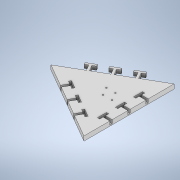
# Autodesk Inventor part: Base2
Saved by Autodesk Inventor 2022.3 (Build 263350000, 350)
## iProperties
Created: 2023-03-28
Part Number: Base2
Material: Generic
Document SubType Name: Modeling
Designer: Manuel Hueso Béjar
Density: 1 g/cm^3
Appearance: Default
Author: Manuel Hueso Béjar
Autodesk Inventor part; units mm, degrees
ref_plane "YZ Plane" through (0, 0, 0) normal (1, 0, 0) x (0, 1, 0)
ref_plane "XZ Plane" through (0, 0, 0) normal (0, 1, 0) x (-1, 0, 0)
ref_plane "XY Plane" through (0, 0, 0) normal (0, 0, 1) x (1, 0, 0)
sketch "Sketch1" plane through (0, 0, 0) normal (0, 1, 0) x (-1, 0, 0)
  circle A0 centre (0, 0) radius 115.470054
  line L0 (115.470054, 0) -> (-57.735027, -100)
  line L1 (-57.735027, -100) -> (-57.735027, 100)
  line L2 (-57.735027, 100) -> (115.470054, 0)
  line L3 (-40.235027, 2.5) -> (-75.235027, 2.5)
  line L4 (-75.235027, 2.5) -> (-75.235027, -2.5)
  line L5 (-75.235027, -2.5) -> (-40.235027, -2.5)
  line L6 (-40.235027, -2.5) -> (-40.235027, 2.5)
  line L7 (-40.235027, 2.5) -> (-75.235027, -2.5) construction
  line L8 (-75.235027, 2.5) -> (-40.235027, -2.5) construction
  line L9 (-42.735027, 10) -> (-37.735027, 10)
  line L10 (-37.735027, 10) -> (-37.735027, -10)
  line L11 (-37.735027, -10) -> (-42.735027, -10)
  line L12 (-42.735027, -10) -> (-42.735027, 10)
  line L13 (-42.735027, 10) -> (-37.735027, -10) construction
  line L14 (-37.735027, 10) -> (-42.735027, -10) construction
  line L15 (-37.735027, 50) -> (-37.735027, 30)
  line L16 (-42.735027, 50) -> (-37.735027, 50)
  line L17 (-42.735027, 30) -> (-42.735027, 50)
  line L18 (-37.735027, 30) -> (-42.735027, 30)
  line L19 (-40.235027, 42.5) -> (-75.235027, 42.5)
  line L20 (-75.235027, 37.5) -> (-40.235027, 37.5)
  line L21 (-37.735027, 90) -> (-37.735027, 70)
  line L22 (-42.735027, 90) -> (-37.735027, 90)
  line L23 (-42.735027, 70) -> (-42.735027, 90)
  line L24 (-37.735027, 70) -> (-42.735027, 70)
  line L25 (-40.235027, 82.5) -> (-75.235027, 82.5)
  line L26 (-75.235027, 77.5) -> (-40.235027, 77.5)
  line L27 (-37.735027, -30) -> (-37.735027, -50)
  line L28 (-42.735027, -30) -> (-37.735027, -30)
  line L29 (-42.735027, -50) -> (-42.735027, -30)
  line L30 (-37.735027, -50) -> (-42.735027, -50)
  line L31 (-40.235027, -37.5) -> (-75.235027, -37.5)
  line L32 (-75.235027, -42.5) -> (-40.235027, -42.5)
  line L33 (-37.735027, 10) -> (-37.735027, -10)
  line L34 (-42.735027, 10) -> (-37.735027, 10)
  line L35 (-42.735027, -10) -> (-42.735027, 10)
  line L36 (-37.735027, -10) -> (-42.735027, -10)
  line L37 (-40.235027, 2.5) -> (-75.235027, 2.5)
  line L38 (-75.235027, -2.5) -> (-40.235027, -2.5)
  line L39 (-37.735027, 50) -> (-37.735027, 30)
  line L40 (-42.735027, 50) -> (-37.735027, 50)
  line L41 (-42.735027, 30) -> (-42.735027, 50)
  line L42 (-37.735027, 30) -> (-42.735027, 30)
  line L43 (-40.235027, 42.5) -> (-75.235027, 42.5)
  line L44 (-75.235027, 37.5) -> (-40.235027, 37.5)
  line L45 (-37.735027, -70) -> (-37.735027, -90)
  line L46 (-42.735027, -70) -> (-37.735027, -70)
  line L47 (-42.735027, -90) -> (-42.735027, -70)
  line L48 (-37.735027, -90) -> (-42.735027, -90)
  line L49 (-40.235027, -77.5) -> (-75.235027, -77.5)
  line L50 (-75.235027, -82.5) -> (-40.235027, -82.5)
  line L51 (-37.735027, -30) -> (-37.735027, -50)
  line L52 (-42.735027, -30) -> (-37.735027, -30)
  line L53 (-42.735027, -50) -> (-42.735027, -30)
  line L54 (-37.735027, -50) -> (-42.735027, -50)
  line L55 (-40.235027, -37.5) -> (-75.235027, -37.5)
  line L56 (-75.235027, -42.5) -> (-40.235027, -42.5)
  line L57 (-37.735027, 10) -> (-37.735027, -10)
  line L58 (-42.735027, 10) -> (-37.735027, 10)
  line L59 (-42.735027, -10) -> (-42.735027, 10)
  line L60 (-37.735027, -10) -> (-42.735027, -10)
  line L61 (-40.235027, 2.5) -> (-75.235027, 2.5)
  line L62 (-75.235027, -2.5) -> (-40.235027, -2.5)
  point P0 (-57.735027, 0)
  point P1 (-40.235027, 0)
  point P2 (-42.735027, 42.5)
  point P3 (-57.735027, 42.5)
  point P4 (-57.735027, 37.5)
  point P5 (-42.735027, 37.5)
  point P6 (-42.735027, -37.5)
  point P7 (-57.735027, -37.5)
  point P8 (-57.735027, -42.5)
  point P9 (-42.735027, -42.5)
  point P10 (-42.735027, 82.5)
  point P11 (-57.735027, 82.5)
  point P12 (-57.735027, 77.5)
  point P13 (-42.735027, 77.5)
  point P14 (-42.735027, -77.5)
  point P15 (-57.735027, -77.5)
  point P16 (-57.735027, -82.5)
  point P17 (-42.735027, -82.5)
  point P18 (-42.735027, -2.5)
  point P19 (-42.735027, 2.5)
  point P20 (-57.735027, 2.5)
  point P21 (-57.735027, -2.5)
  point P22 (-40.414519, -90)
  point P23 (-37.735027, -88.452995)
  point P24 (-37.735027, 88.452995)
  point P25 (-40.414519, 90)
  dimension "d1" = 200
  dimension "d2" = 35
  dimension "d3" = 5
  dimension "d4" = 5
  dimension "d5" = 20
  dimension "d8" = 40
  dimension "d11" = 40
  constraints: 126 end point, 6 midpoint, 4 parallel, 2 coincident, 2 horizontal, 2 perpendicular, 2 vertical, 1 horizontal alignment, 121 other
  measures "d1" distance of L0.end L1.end
  measures "d2" distance of L5.end L4.end
  measures "d3" distance of L4.end L3.end
  measures "d4" distance of L10.end L11.end
  measures "d5" distance of L9.end L10.end
  measures "d8" distance of L9.end L15.start
  measures "d11" distance of L9.end L27.start
sketch "Sketch1 outline for Extrusion1" plane through (0, 0, 0) normal (0, 1, 0) x (-1, 0, 0)
  line L0 (-57.735027, 100) -> (-57.735027, -100)
  line L1 (115.470054, 0) -> (-57.735027, 100)
  line L2 (-57.735027, -100) -> (115.470054, 0)
extrude "Extrusion1" add sketch "Sketch1 outline for Extrusion1" along normal blind 10
sketch "Sketch1 outline for Extrusion2" plane through (0, 0, 0) normal (0, 1, 0) x (-1, 0, 0)
  line L0 (-42.735027, 30) -> (-37.735027, 30)
  line L1 (-42.735027, 37.5) -> (-42.735027, 30)
  line L2 (-57.735027, 37.5) -> (-42.735027, 37.5)
  line L3 (-57.735027, 42.5) -> (-57.735027, 37.5)
  line L4 (-42.735027, 42.5) -> (-57.735027, 42.5)
  line L5 (-42.735027, 50) -> (-42.735027, 42.5)
  line L6 (-37.735027, 50) -> (-42.735027, 50)
  line L7 (-37.735027, 30) -> (-37.735027, 50)
  line L8 (-42.735027, -50) -> (-37.735027, -50)
  line L9 (-42.735027, -42.5) -> (-42.735027, -50)
  line L10 (-57.735027, -42.5) -> (-42.735027, -42.5)
  line L11 (-57.735027, -37.5) -> (-57.735027, -42.5)
  line L12 (-42.735027, -37.5) -> (-57.735027, -37.5)
  line L13 (-42.735027, -30) -> (-42.735027, -37.5)
  line L14 (-37.735027, -30) -> (-42.735027, -30)
  line L15 (-37.735027, -50) -> (-37.735027, -30)
  line L16 (-42.735027, -2.5) -> (-42.735027, -10)
  line L17 (-57.735027, -2.5) -> (-42.735027, -2.5)
  line L18 (-57.735027, 2.5) -> (-57.735027, -2.5)
  line L19 (-42.735027, 2.5) -> (-57.735027, 2.5)
  line L20 (-42.735027, 10) -> (-42.735027, 2.5)
  line L21 (-37.735027, 10) -> (-42.735027, 10)
  line L22 (-37.735027, -10) -> (-37.735027, 10)
  line L23 (-42.735027, -10) -> (-37.735027, -10)
extrude "Extrusion2" cut sketch "Sketch1 outline for Extrusion2" along normal blind 10
sketch "Sketch1 outline for Extrusion3" plane through (0, 0, 0) normal (0, 1, 0) x (-1, 0, 0)
  line L0 (-42.735027, 30) -> (-37.735027, 30)
  line L1 (-42.735027, 37.5) -> (-42.735027, 30)
  line L2 (-57.735027, 37.5) -> (-42.735027, 37.5)
  line L3 (-57.735027, 42.5) -> (-57.735027, 37.5)
  line L4 (-42.735027, 42.5) -> (-57.735027, 42.5)
  line L5 (-42.735027, 50) -> (-42.735027, 42.5)
  line L6 (-37.735027, 50) -> (-42.735027, 50)
  line L7 (-37.735027, 30) -> (-37.735027, 50)
  line L8 (-42.735027, -50) -> (-37.735027, -50)
  line L9 (-42.735027, -42.5) -> (-42.735027, -50)
  line L10 (-57.735027, -42.5) -> (-42.735027, -42.5)
  line L11 (-57.735027, -37.5) -> (-57.735027, -42.5)
  line L12 (-42.735027, -37.5) -> (-57.735027, -37.5)
  line L13 (-42.735027, -30) -> (-42.735027, -37.5)
  line L14 (-37.735027, -30) -> (-42.735027, -30)
  line L15 (-37.735027, -50) -> (-37.735027, -30)
  line L16 (-42.735027, -2.5) -> (-42.735027, -10)
  line L17 (-57.735027, -2.5) -> (-42.735027, -2.5)
  line L18 (-57.735027, 2.5) -> (-57.735027, -2.5)
  line L19 (-42.735027, 2.5) -> (-57.735027, 2.5)
  line L20 (-42.735027, 10) -> (-42.735027, 2.5)
  line L21 (-37.735027, 10) -> (-42.735027, 10)
  line L22 (-37.735027, -10) -> (-37.735027, 10)
  line L23 (-42.735027, -10) -> (-37.735027, -10)
  line L24 (-37.735027, -70) -> (-42.735027, -70)
  line L25 (-37.735027, -88.452995) -> (-37.735027, -70)
  line L26 (-40.414519, -90) -> (-37.735027, -88.452995)
  line L27 (-42.735027, -90) -> (-40.414519, -90)
  line L28 (-42.735027, -82.5) -> (-42.735027, -90)
  line L29 (-57.735027, -82.5) -> (-42.735027, -82.5)
  line L30 (-57.735027, -77.5) -> (-57.735027, -82.5)
  line L31 (-42.735027, -77.5) -> (-57.735027, -77.5)
  line L32 (-42.735027, -70) -> (-42.735027, -77.5)
  line L33 (-42.735027, 70) -> (-37.735027, 70)
  line L34 (-42.735027, 77.5) -> (-42.735027, 70)
  line L35 (-57.735027, 77.5) -> (-42.735027, 77.5)
  line L36 (-57.735027, 82.5) -> (-57.735027, 77.5)
  line L37 (-42.735027, 82.5) -> (-57.735027, 82.5)
  line L38 (-42.735027, 90) -> (-42.735027, 82.5)
  line L39 (-40.414519, 90) -> (-42.735027, 90)
  line L40 (-37.735027, 88.452995) -> (-40.414519, 90)
  line L41 (-37.735027, 70) -> (-37.735027, 88.452995)
extrude "Extrusion3" add sketch "Sketch1 outline for Extrusion3" along normal blind 2.2
sketch "Sketch2" plane through (0, 0, 0) normal (0, -1, 0) x (1, 0, 0)
  line L0 (57.735027, 100) -> (57.735027, -100)
  line L1 (-115.470054, 0) -> (57.735027, 100)
  line L2 (57.735027, -100) -> (-115.470054, 0)
  line L3 (35.735027, 61.894882) -> (35.735027, -61.894882)
  line L4 (35.735027, -61.894882) -> (-71.470054, 0)
  line L5 (-71.470054, 0) -> (35.735027, 61.894882)
  line L6 (32.735027, 56.69873) -> (32.735027, -56.69873)
  line L7 (32.735027, -56.69873) -> (-65.470054, 0)
  line L8 (-65.470054, 0) -> (32.735027, 56.69873)
  point P0 (0, 0)
  dimension "d20" = 22
  dimension "d21" = 3
  constraints: 12 end point, 4 other
  measures "d20" distance between parallel lines of L1 L5
  measures "d21" distance between parallel lines of L5 L8
sketch "Sketch2 outline for Extrusion4" plane through (0, 0, 0) normal (0, -1, 0) x (1, 0, 0)
  line L0 (35.735027, 61.894882) -> (-71.470054, 0)
  line L1 (35.735027, -61.894882) -> (35.735027, 61.894882)
  line L2 (-71.470054, 0) -> (35.735027, -61.894882)
  line L3 (32.735027, 56.69873) -> (32.735027, -56.69873)
  line L4 (-65.470054, 0) -> (32.735027, 56.69873)
  line L5 (32.735027, -56.69873) -> (-65.470054, 0)
extrude "Extrusion4" cut sketch "Sketch2 outline for Extrusion4" against normal blind 1.5
sketch "Sketch3" plane through (0, 10, 0) normal (0, 1, 0) x (1, 0, 0)
  line L0 (57.735027, 100) -> (-115.470054, 0)
  line L1 (-28.867513, 50) -> (-36.367513, 62.990381)
  line L2 (-28.867513, 50) -> (-13.867513, 50) construction
  line L3 (-34.20245, 64.240381) -> (-27.707259, 67.990381)
  line L4 (-27.707259, 67.990381) -> (-30.207259, 72.320508)
  line L5 (-30.207259, 72.320508) -> (-47.527767, 62.320508)
  line L6 (-47.527767, 62.320508) -> (-45.027767, 57.990381)
  line L7 (-45.027767, 57.990381) -> (-38.532577, 61.740381)
  line L8 (-28.867513, 50) -> (-31.032577, 48.75)
  line L9 (-31.032577, 48.75) -> (-38.532577, 61.740381)
  line L10 (-31.032577, 48.75) -> (-26.70245, 51.25)
  line L11 (-26.70245, 51.25) -> (-34.20245, 64.240381)
  line L12 (-28.867513, -50) -> (-36.367513, -37.009619) construction
  line L13 (-28.867513, -50) -> (-26.70245, -51.25)
  line L14 (-26.70245, -51.25) -> (-31.032577, -48.75)
  line L15 (-28.867513, -50) -> (-36.367513, -62.990381)
  line L16 (-26.70245, -51.25) -> (-34.20245, -64.240381)
  line L17 (-31.032577, -48.75) -> (-38.532577, -61.740381)
  line L18 (-38.532577, -61.740381) -> (-45.027767, -57.990381)
  line L19 (-27.707259, -67.990381) -> (-34.20245, -64.240381)
  line L20 (-45.027767, -57.990381) -> (-47.527767, -62.320508)
  line L21 (-30.207259, -72.320508) -> (-27.707259, -67.990381)
  line L22 (-47.527767, -62.320508) -> (-30.207259, -72.320508)
  line L23 (-82.168784, 42.320508) -> (-79.668784, 37.990381)
  line L24 (-79.668784, 37.990381) -> (-73.173593, 41.740381)
  line L25 (-63.50853, 30) -> (-65.673593, 28.75)
  line L26 (-65.673593, 28.75) -> (-61.343466, 31.25)
  line L27 (-65.673593, 28.75) -> (-73.173593, 41.740381)
  line L28 (-63.50853, 30) -> (-71.00853, 42.990381)
  line L29 (-61.343466, 31.25) -> (-68.843466, 44.240381)
  line L30 (-64.848276, 52.320508) -> (-82.168784, 42.320508)
  line L31 (-63.50853, 30) -> (-48.50853, 30) construction
  line L32 (-62.348276, 47.990381) -> (-64.848276, 52.320508)
  line L33 (-68.843466, 44.240381) -> (-62.348276, 47.990381)
  line L34 (-116.8098, 22.320508) -> (-114.3098, 17.990381)
  line L35 (-114.3098, 17.990381) -> (-107.814609, 21.740381)
  line L36 (-98.149546, 10) -> (-100.314609, 8.75)
  line L37 (-100.314609, 8.75) -> (-95.984482, 11.25)
  line L38 (-100.314609, 8.75) -> (-107.814609, 21.740381)
  line L39 (-98.149546, 10) -> (-105.649546, 22.990381)
  line L40 (-95.984482, 11.25) -> (-103.484482, 24.240381)
  line L41 (-99.489292, 32.320508) -> (-116.8098, 22.320508)
  line L42 (-98.149546, 10) -> (-83.149546, 10) construction
  line L43 (-96.989292, 27.990381) -> (-99.489292, 32.320508)
  line L44 (-103.484482, 24.240381) -> (-96.989292, 27.990381)
  line L45 (-12.886751, 82.320508) -> (-10.386751, 77.990381)
  line L46 (-10.386751, 77.990381) -> (-3.891561, 81.740381)
  line L47 (5.773503, 70) -> (3.608439, 68.75)
  line L48 (3.608439, 68.75) -> (7.938566, 71.25)
  line L49 (3.608439, 68.75) -> (-3.891561, 81.740381)
  line L50 (5.773503, 70) -> (-1.726497, 82.990381)
  line L51 (7.938566, 71.25) -> (0.438566, 84.240381)
  line L52 (4.433757, 92.320508) -> (-12.886751, 82.320508)
  line L53 (5.773503, 70) -> (20.773503, 70) construction
  line L54 (6.933757, 87.990381) -> (4.433757, 92.320508)
  line L55 (0.438566, 84.240381) -> (6.933757, 87.990381)
  line L56 (-47.527767, 62.320508) -> (-45.027767, 57.990381)
  line L57 (-45.027767, 57.990381) -> (-38.532577, 61.740381)
  line L58 (-28.867513, 50) -> (-31.032577, 48.75)
  line L59 (-31.032577, 48.75) -> (-26.70245, 51.25)
  line L60 (-31.032577, 48.75) -> (-38.532577, 61.740381)
  line L61 (-28.867513, 50) -> (-36.367513, 62.990381)
  line L62 (-26.70245, 51.25) -> (-34.20245, 64.240381)
  line L63 (-30.207259, 72.320508) -> (-47.527767, 62.320508)
  line L64 (-28.867513, 50) -> (-13.867513, 50) construction
  line L65 (-27.707259, 67.990381) -> (-30.207259, 72.320508)
  line L66 (-34.20245, 64.240381) -> (-27.707259, 67.990381)
  line L67 (-82.168784, 42.320508) -> (-79.668784, 37.990381)
  line L68 (-79.668784, 37.990381) -> (-73.173593, 41.740381)
  line L69 (-63.50853, 30) -> (-65.673593, 28.75)
  line L70 (-65.673593, 28.75) -> (-61.343466, 31.25)
  line L71 (-65.673593, 28.75) -> (-73.173593, 41.740381)
  line L72 (-63.50853, 30) -> (-71.00853, 42.990381)
  line L73 (-61.343466, 31.25) -> (-68.843466, 44.240381)
  line L74 (-64.848276, 52.320508) -> (-82.168784, 42.320508)
  line L75 (-63.50853, 30) -> (-48.50853, 30) construction
  line L76 (-62.348276, 47.990381) -> (-64.848276, 52.320508)
  line L77 (-68.843466, 44.240381) -> (-62.348276, 47.990381)
  line L78 (21.754265, 102.320508) -> (24.254265, 97.990381)
  line L79 (24.254265, 97.990381) -> (30.749455, 101.740381)
  line L80 (40.414519, 90) -> (38.249455, 88.75)
  line L81 (38.249455, 88.75) -> (42.579582, 91.25)
  line L82 (38.249455, 88.75) -> (30.749455, 101.740381)
  line L83 (40.414519, 90) -> (32.914519, 102.990381)
  line L84 (42.579582, 91.25) -> (35.079582, 104.240381)
  line L85 (39.074773, 112.320508) -> (21.754265, 102.320508)
  line L86 (40.414519, 90) -> (55.414519, 90) construction
  line L87 (41.574773, 107.990381) -> (39.074773, 112.320508)
  line L88 (35.079582, 104.240381) -> (41.574773, 107.990381)
  line L89 (-12.886751, 82.320508) -> (-10.386751, 77.990381)
  line L90 (-10.386751, 77.990381) -> (-3.891561, 81.740381)
  line L91 (5.773503, 70) -> (3.608439, 68.75)
  line L92 (3.608439, 68.75) -> (7.938566, 71.25)
  line L93 (3.608439, 68.75) -> (-3.891561, 81.740381)
  line L94 (5.773503, 70) -> (-1.726497, 82.990381)
  line L95 (7.938566, 71.25) -> (0.438566, 84.240381)
  line L96 (4.433757, 92.320508) -> (-12.886751, 82.320508)
  line L97 (5.773503, 70) -> (20.773503, 70) construction
  line L98 (6.933757, 87.990381) -> (4.433757, 92.320508)
  line L99 (0.438566, 84.240381) -> (6.933757, 87.990381)
  line L100 (-47.527767, 62.320508) -> (-45.027767, 57.990381)
  line L101 (-45.027767, 57.990381) -> (-38.532577, 61.740381)
  line L102 (-28.867513, 50) -> (-31.032577, 48.75)
  line L103 (-31.032577, 48.75) -> (-26.70245, 51.25)
  line L104 (-31.032577, 48.75) -> (-38.532577, 61.740381)
  line L105 (-28.867513, 50) -> (-36.367513, 62.990381)
  line L106 (-26.70245, 51.25) -> (-34.20245, 64.240381)
  line L107 (-30.207259, 72.320508) -> (-47.527767, 62.320508)
  line L108 (-28.867513, 50) -> (-13.867513, 50) construction
  line L109 (-27.707259, 67.990381) -> (-30.207259, 72.320508)
  line L110 (-34.20245, 64.240381) -> (-27.707259, 67.990381)
  line L111 (-115.470054, 0) -> (57.735027, -100)
  line L112 (57.735027, -100) -> (-115.470054, 0)
  line L113 (5.773503, -70) -> (-1.726497, -57.009619) construction
  line L114 (5.773503, -70) -> (7.938566, -71.25)
  line L115 (7.938566, -71.25) -> (3.608439, -68.75)
  line L116 (3.608439, -68.75) -> (-3.891561, -81.740381)
  line L117 (5.773503, -70) -> (-1.726497, -82.990381)
  line L118 (7.938566, -71.25) -> (0.438566, -84.240381)
  line L119 (-3.891561, -81.740381) -> (-10.386751, -77.990381)
  line L120 (-10.386751, -77.990381) -> (-12.886751, -82.320508)
  line L121 (6.933757, -87.990381) -> (0.438566, -84.240381)
  line L122 (4.433757, -92.320508) -> (6.933757, -87.990381)
  line L123 (-12.886751, -82.320508) -> (4.433757, -92.320508)
  line L124 (40.414519, -90) -> (32.914519, -77.009619) construction
  line L125 (40.414519, -90) -> (42.579582, -91.25)
  line L126 (42.579582, -91.25) -> (38.249455, -88.75)
  line L127 (38.249455, -88.75) -> (30.749455, -101.740381)
  line L128 (40.414519, -90) -> (32.914519, -102.990381)
  line L129 (42.579582, -91.25) -> (35.079582, -104.240381)
  line L130 (30.749455, -101.740381) -> (24.254265, -97.990381)
  line L131 (24.254265, -97.990381) -> (21.754265, -102.320508)
  line L132 (41.574773, -107.990381) -> (35.079582, -104.240381)
  line L133 (39.074773, -112.320508) -> (41.574773, -107.990381)
  line L134 (21.754265, -102.320508) -> (39.074773, -112.320508)
  line L135 (-63.50853, -30) -> (-71.00853, -17.009619) construction
  line L136 (-63.50853, -30) -> (-61.343466, -31.25)
  line L137 (-61.343466, -31.25) -> (-65.673593, -28.75)
  line L138 (-65.673593, -28.75) -> (-73.173593, -41.740381)
  line L139 (-63.50853, -30) -> (-71.00853, -42.990381)
  line L140 (-61.343466, -31.25) -> (-68.843466, -44.240381)
  line L141 (-73.173593, -41.740381) -> (-79.668784, -37.990381)
  line L142 (-79.668784, -37.990381) -> (-82.168784, -42.320508)
  line L143 (-62.348276, -47.990381) -> (-68.843466, -44.240381)
  line L144 (-64.848276, -52.320508) -> (-62.348276, -47.990381)
  line L145 (-82.168784, -42.320508) -> (-64.848276, -52.320508)
  line L146 (-28.867513, -50) -> (-36.367513, -37.009619) construction
  line L147 (-28.867513, -50) -> (-26.70245, -51.25)
  line L148 (-26.70245, -51.25) -> (-31.032577, -48.75)
  line L149 (-31.032577, -48.75) -> (-38.532577, -61.740381)
  line L150 (-28.867513, -50) -> (-36.367513, -62.990381)
  line L151 (-26.70245, -51.25) -> (-34.20245, -64.240381)
  line L152 (-38.532577, -61.740381) -> (-45.027767, -57.990381)
  line L153 (-45.027767, -57.990381) -> (-47.527767, -62.320508)
  line L154 (-27.707259, -67.990381) -> (-34.20245, -64.240381)
  line L155 (-30.207259, -72.320508) -> (-27.707259, -67.990381)
  line L156 (-47.527767, -62.320508) -> (-30.207259, -72.320508)
  line L157 (5.773503, -70) -> (-1.726497, -57.009619) construction
  line L158 (5.773503, -70) -> (7.938566, -71.25)
  line L159 (7.938566, -71.25) -> (3.608439, -68.75)
  line L160 (3.608439, -68.75) -> (-3.891561, -81.740381)
  line L161 (5.773503, -70) -> (-1.726497, -82.990381)
  line L162 (7.938566, -71.25) -> (0.438566, -84.240381)
  line L163 (-3.891561, -81.740381) -> (-10.386751, -77.990381)
  line L164 (-10.386751, -77.990381) -> (-12.886751, -82.320508)
  line L165 (6.933757, -87.990381) -> (0.438566, -84.240381)
  line L166 (4.433757, -92.320508) -> (6.933757, -87.990381)
  line L167 (-12.886751, -82.320508) -> (4.433757, -92.320508)
  line L168 (-98.149546, -10) -> (-105.649546, 2.990381) construction
  line L169 (-98.149546, -10) -> (-95.984482, -11.25)
  line L170 (-95.984482, -11.25) -> (-100.314609, -8.75)
  line L171 (-100.314609, -8.75) -> (-107.814609, -21.740381)
  line L172 (-98.149546, -10) -> (-105.649546, -22.990381)
  line L173 (-95.984482, -11.25) -> (-103.484482, -24.240381)
  line L174 (-107.814609, -21.740381) -> (-114.3098, -17.990381)
  line L175 (-114.3098, -17.990381) -> (-116.8098, -22.320508)
  line L176 (-96.989292, -27.990381) -> (-103.484482, -24.240381)
  line L177 (-99.489292, -32.320508) -> (-96.989292, -27.990381)
  line L178 (-116.8098, -22.320508) -> (-99.489292, -32.320508)
  line L179 (-63.50853, -30) -> (-71.00853, -17.009619) construction
  line L180 (-63.50853, -30) -> (-61.343466, -31.25)
  line L181 (-61.343466, -31.25) -> (-65.673593, -28.75)
  line L182 (-65.673593, -28.75) -> (-73.173593, -41.740381)
  line L183 (-63.50853, -30) -> (-71.00853, -42.990381)
  line L184 (-61.343466, -31.25) -> (-68.843466, -44.240381)
  line L185 (-73.173593, -41.740381) -> (-79.668784, -37.990381)
  line L186 (-79.668784, -37.990381) -> (-82.168784, -42.320508)
  line L187 (-62.348276, -47.990381) -> (-68.843466, -44.240381)
  line L188 (-64.848276, -52.320508) -> (-62.348276, -47.990381)
  line L189 (-82.168784, -42.320508) -> (-64.848276, -52.320508)
  line L190 (-28.867513, -50) -> (-36.367513, -37.009619) construction
  line L191 (-28.867513, -50) -> (-26.70245, -51.25)
  line L192 (-26.70245, -51.25) -> (-31.032577, -48.75)
  line L193 (-31.032577, -48.75) -> (-38.532577, -61.740381)
  line L194 (-28.867513, -50) -> (-36.367513, -62.990381)
  line L195 (-26.70245, -51.25) -> (-34.20245, -64.240381)
  line L196 (-38.532577, -61.740381) -> (-45.027767, -57.990381)
  line L197 (-45.027767, -57.990381) -> (-47.527767, -62.320508)
  line L198 (-27.707259, -67.990381) -> (-34.20245, -64.240381)
  line L199 (-30.207259, -72.320508) -> (-27.707259, -67.990381)
  line L200 (-47.527767, -62.320508) -> (-30.207259, -72.320508)
  line L201 (-28.867513, -50) -> (-43.867513, -50) construction
  line L202 (-28.867513, -50) -> (-21.367513, -37.009619)
  line L203 (-26.70245, -51.25) -> (-19.20245, -38.259619)
  line L204 (-31.032577, -48.75) -> (-23.532577, -35.759619)
  line L205 (-23.532577, -35.759619) -> (-30.027767, -32.009619)
  line L206 (-12.707259, -42.009619) -> (-19.20245, -38.259619)
  line L207 (-30.027767, -32.009619) -> (-27.527767, -27.679492)
  line L208 (-10.207259, -37.679492) -> (-12.707259, -42.009619)
  line L209 (-27.527767, -27.679492) -> (-10.207259, -37.679492)
  line L210 (5.773503, -70) -> (-9.226497, -70) construction
  line L211 (3.608439, -68.75) -> (11.108439, -55.759619)
  line L212 (5.773503, -70) -> (13.273503, -57.009619)
  line L213 (7.938566, -71.25) -> (15.438566, -58.259619)
  line L214 (11.108439, -55.759619) -> (4.613249, -52.009619)
  line L215 (4.613249, -52.009619) -> (7.113249, -47.679492)
  line L216 (21.933757, -62.009619) -> (15.438566, -58.259619)
  line L217 (24.433757, -57.679492) -> (21.933757, -62.009619)
  line L218 (7.113249, -47.679492) -> (24.433757, -57.679492)
  line L219 (40.414519, -90) -> (25.414519, -90) construction
  line L220 (38.249455, -88.75) -> (45.749455, -75.759619)
  line L221 (40.414519, -90) -> (47.914519, -77.009619)
  line L222 (42.579582, -91.25) -> (50.079582, -78.259619)
  line L223 (45.749455, -75.759619) -> (39.254265, -72.009619)
  line L224 (39.254265, -72.009619) -> (41.754265, -67.679492)
  line L225 (56.574773, -82.009619) -> (50.079582, -78.259619)
  line L226 (59.074773, -77.679492) -> (56.574773, -82.009619)
  line L227 (41.754265, -67.679492) -> (59.074773, -77.679492)
  line L228 (-63.50853, -30) -> (-78.50853, -30) construction
  line L229 (-65.673593, -28.75) -> (-58.173593, -15.759619)
  line L230 (-63.50853, -30) -> (-56.00853, -17.009619)
  line L231 (-61.343466, -31.25) -> (-53.843466, -18.259619)
  line L232 (-58.173593, -15.759619) -> (-64.668784, -12.009619)
  line L233 (-64.668784, -12.009619) -> (-62.168784, -7.679492)
  line L234 (-47.348276, -22.009619) -> (-53.843466, -18.259619)
  line L235 (-44.848276, -17.679492) -> (-47.348276, -22.009619)
  line L236 (-62.168784, -7.679492) -> (-44.848276, -17.679492)
  line L237 (-28.867513, -50) -> (-43.867513, -50) construction
  line L238 (-31.032577, -48.75) -> (-23.532577, -35.759619)
  line L239 (-28.867513, -50) -> (-21.367513, -37.009619)
  line L240 (-26.70245, -51.25) -> (-19.20245, -38.259619)
  line L241 (-23.532577, -35.759619) -> (-30.027767, -32.009619)
  line L242 (-30.027767, -32.009619) -> (-27.527767, -27.679492)
  line L243 (-12.707259, -42.009619) -> (-19.20245, -38.259619)
  line L244 (-10.207259, -37.679492) -> (-12.707259, -42.009619)
  line L245 (-27.527767, -27.679492) -> (-10.207259, -37.679492)
  line L246 (5.773503, -70) -> (-9.226497, -70) construction
  line L247 (3.608439, -68.75) -> (11.108439, -55.759619)
  line L248 (5.773503, -70) -> (13.273503, -57.009619)
  line L249 (7.938566, -71.25) -> (15.438566, -58.259619)
  line L250 (11.108439, -55.759619) -> (4.613249, -52.009619)
  line L251 (4.613249, -52.009619) -> (7.113249, -47.679492)
  line L252 (21.933757, -62.009619) -> (15.438566, -58.259619)
  line L253 (24.433757, -57.679492) -> (21.933757, -62.009619)
  line L254 (7.113249, -47.679492) -> (24.433757, -57.679492)
  line L255 (-98.149546, -10) -> (-113.149546, -10) construction
  line L256 (-100.314609, -8.75) -> (-92.814609, 4.240381)
  line L257 (-98.149546, -10) -> (-90.649546, 2.990381)
  line L258 (-95.984482, -11.25) -> (-88.484482, 1.740381)
  line L259 (-92.814609, 4.240381) -> (-99.3098, 7.990381)
  line L260 (-99.3098, 7.990381) -> (-96.8098, 12.320508)
  line L261 (-81.989292, -2.009619) -> (-88.484482, 1.740381)
  line L262 (-79.489292, 2.320508) -> (-81.989292, -2.009619)
  line L263 (-96.8098, 12.320508) -> (-79.489292, 2.320508)
  line L264 (-63.50853, -30) -> (-78.50853, -30) construction
  line L265 (-65.673593, -28.75) -> (-58.173593, -15.759619)
  line L266 (-63.50853, -30) -> (-56.00853, -17.009619)
  line L267 (-61.343466, -31.25) -> (-53.843466, -18.259619)
  line L268 (-58.173593, -15.759619) -> (-64.668784, -12.009619)
  line L269 (-64.668784, -12.009619) -> (-62.168784, -7.679492)
  line L270 (-47.348276, -22.009619) -> (-53.843466, -18.259619)
  line L271 (-44.848276, -17.679492) -> (-47.348276, -22.009619)
  line L272 (-62.168784, -7.679492) -> (-44.848276, -17.679492)
  line L273 (-28.867513, -50) -> (-43.867513, -50) construction
  line L274 (-31.032577, -48.75) -> (-23.532577, -35.759619)
  line L275 (-28.867513, -50) -> (-21.367513, -37.009619)
  line L276 (-26.70245, -51.25) -> (-19.20245, -38.259619)
  line L277 (-23.532577, -35.759619) -> (-30.027767, -32.009619)
  line L278 (-30.027767, -32.009619) -> (-27.527767, -27.679492)
  line L279 (-12.707259, -42.009619) -> (-19.20245, -38.259619)
  line L280 (-10.207259, -37.679492) -> (-12.707259, -42.009619)
  line L281 (-27.527767, -27.679492) -> (-10.207259, -37.679492)
  point P0 (0, 0)
  point P1 (3.608439, 68.75)
  point P2 (7.938566, 71.25)
  point P3 (-65.673593, 28.75)
  point P4 (-61.343466, 31.25)
  point P5 (-100.314609, 8.75)
  point P6 (-95.984482, 11.25)
  point P7 (42.579582, -91.25)
  point P8 (38.249455, -88.75)
  point P9 (7.938566, -71.25)
  point P10 (3.608439, -68.75)
  point P11 (-61.343466, -31.25)
  point P12 (-65.673593, -28.75)
  point P13 (-95.984482, -11.25)
  point P14 (-100.314609, -8.75)
  point P15 (7.938566, -71.25)
  point P16 (3.608439, -68.75)
  point P17 (-12.707259, -42.009619)
  point P18 (-65.673593, -28.75)
  point P19 (-61.343466, -31.25)
  dimension "d24" = 15
  dimension "d25" = 120
  dimension "d26" = 10
  dimension "d27" = 5
  dimension "d28" = 20
  dimension "d29" = 90
  dimension "d30" = 5
  dimension "d31" = 2.5
  dimension "d32" = 5
  dimension "d35" = 120
  dimension "d39" = 40
  dimension "d42" = 40
  dimension "d47" = 40
  dimension "d50" = 40
  constraints: 560 end point, 72 symmetric about line, 6 perpendicular, 2 point on line, 1 collinear, 1 equal length, 1 horizontal, 1 midpoint, 379 other
  measures "d24" distance of L1.start L1.end
  measures "d25" angle of L2 L1
  measures "d26" distance of L1.end L3.end
  measures "d27" distance of L3.end L4.end
  measures "d28" distance of L4.end L5.end
  measures "d29" angle of L5 L4
  measures "d30" distance of L5.end L6.end
  measures "d31" distance of L1.start L8.end
  measures "d32" distance of L8.end L10.end
  measures "d39" distance of L6.end L23.end
  measures "d42" distance of L6.end L45.end
  measures "d47" distance of L12.end L113.end
  measures "d50" distance of L12.end L135.end
sketch "Sketch3 outline for Extrusion6" plane through (0, 10, 0) normal (0, 1, 0) x (1, 0, 0)
  line L0 (7.938566, -71.25) -> (15.438566, -58.259619)
  line L1 (3.608439, -68.75) -> (7.938566, -71.25)
  line L2 (11.108439, -55.759619) -> (3.608439, -68.75)
  line L3 (4.613249, -52.009619) -> (11.108439, -55.759619)
  line L4 (7.113249, -47.679492) -> (4.613249, -52.009619)
  line L5 (24.433757, -57.679492) -> (7.113249, -47.679492)
  line L6 (21.933757, -62.009619) -> (24.433757, -57.679492)
  line L7 (15.438566, -58.259619) -> (21.933757, -62.009619)
  line L8 (-10.207259, -37.679492) -> (-27.527767, -27.679492)
  line L9 (-27.527767, -27.679492) -> (-30.027767, -32.009619)
  line L10 (-30.027767, -32.009619) -> (-23.532577, -35.759619)
  line L11 (-23.532577, -35.759619) -> (-31.032577, -48.75)
  line L12 (-31.032577, -48.75) -> (-26.70245, -51.25)
  line L13 (-26.70245, -51.25) -> (-19.20245, -38.259619)
  line L14 (-19.20245, -38.259619) -> (-12.707259, -42.009619)
  line L15 (-12.707259, -42.009619) -> (-10.207259, -37.679492)
  line L16 (-44.848276, -17.679492) -> (-62.168784, -7.679492)
  line L17 (-47.348276, -22.009619) -> (-44.848276, -17.679492)
  line L18 (-53.843466, -18.259619) -> (-47.348276, -22.009619)
  line L19 (-61.343466, -31.25) -> (-53.843466, -18.259619)
  line L20 (-65.673593, -28.75) -> (-61.343466, -31.25)
  line L21 (-58.173593, -15.759619) -> (-65.673593, -28.75)
  line L22 (-64.668784, -12.009619) -> (-58.173593, -15.759619)
  line L23 (-62.168784, -7.679492) -> (-64.668784, -12.009619)
extrude "Extrusion6" cut sketch "Sketch3 outline for Extrusion6" against normal blind 7.8
sketch "Sketch3 outline for Extrusion7" plane through (0, 10, 0) normal (0, 1, 0) x (1, 0, 0)
  line L0 (0.438566, 84.240381) -> (6.933757, 87.990381)
  line L1 (7.938566, 71.25) -> (0.438566, 84.240381)
  line L2 (3.608439, 68.75) -> (7.938566, 71.25)
  line L3 (-3.891561, 81.740381) -> (3.608439, 68.75)
  line L4 (-10.386751, 77.990381) -> (-3.891561, 81.740381)
  line L5 (-12.886751, 82.320508) -> (-10.386751, 77.990381)
  line L6 (4.433757, 92.320508) -> (-12.886751, 82.320508)
  line L7 (6.933757, 87.990381) -> (4.433757, 92.320508)
  line L8 (-26.70245, 51.25) -> (-34.20245, 64.240381)
  line L9 (-31.032577, 48.75) -> (-26.70245, 51.25)
  line L10 (-38.532577, 61.740381) -> (-31.032577, 48.75)
  line L11 (-45.027767, 57.990381) -> (-38.532577, 61.740381)
  line L12 (-47.527767, 62.320508) -> (-45.027767, 57.990381)
  line L13 (-30.207259, 72.320508) -> (-47.527767, 62.320508)
  line L14 (-27.707259, 67.990381) -> (-30.207259, 72.320508)
  line L15 (-34.20245, 64.240381) -> (-27.707259, 67.990381)
  line L16 (-68.843466, 44.240381) -> (-62.348276, 47.990381)
  line L17 (-61.343466, 31.25) -> (-68.843466, 44.240381)
  line L18 (-65.673593, 28.75) -> (-61.343466, 31.25)
  line L19 (-73.173593, 41.740381) -> (-65.673593, 28.75)
  line L20 (-79.668784, 37.990381) -> (-73.173593, 41.740381)
  line L21 (-82.168784, 42.320508) -> (-79.668784, 37.990381)
  line L22 (-64.848276, 52.320508) -> (-82.168784, 42.320508)
  line L23 (-62.348276, 47.990381) -> (-64.848276, 52.320508)
extrude "Extrusion7" add sketch "Sketch3 outline for Extrusion7" against normal up to surface (7.8 mm away)
sketch "Sketch4" plane through (0, 10, 0) normal (0, 1, 0) x (1, 0, 0)
  line L0 (-115.470054, 0) -> (57.735027, 0)
  line L1 (57.735027, -100) -> (57.735027, 100)
  line L2 (57.735027, -100) -> (-28.867513, 50)
  line L3 (57.735027, 100) -> (-115.470054, 0)
  line L4 (57.735027, 100) -> (-28.867513, -50)
  line L5 (-115.470054, 0) -> (57.735027, -100)
  circle A0 centre (0, 0) radius 20
  line L6 (10, 17.320508) -> (20, 0)
  line L7 (20, 0) -> (10, -17.320508)
  line L8 (10, -17.320508) -> (-10, -17.320508)
  line L9 (-10, -17.320508) -> (-20, 0)
  line L10 (-20, 0) -> (-10, 17.320508)
  line L11 (-10, 17.320508) -> (10, 17.320508)
  dimension "d59" = 40
  constraints: 18 end point, 3 midpoint, 2 coincident, 1 point on line, 16 other
hole "Hole1" at (0, 10, 0) at (-10, 10, -17.320508) at (20, 10, 0) at (10, 10, -17.320508) direction (0, -1, 0) diameter 2.2 depth 6.3 counterbore diameter 3.1 counterbore depth 4.1
thicken "Thicken1" operation add thickness 0.05 both sides no extend neighbours yes toward (-0.8660254, 0, -0.5) faces at (-60.673593, 4.8, 20.089746) (-62.50372, 7.4, 13.259619) (-63.002117, 7.4, 9.122868) (-50.621778, 7.4, 14.346159) (-46.514942, 7.4, 20.566243) (-51.678403, 7.4, 19.509619) (-58.843466, 4.8, 26.919873)
thicken "Thicken2" operation add thickness 0.05 both sides no extend neighbours yes toward (-0.8660254, 0, -0.5) faces at (-26.032577, 7.4, 40.089746) (-27.862704, 7.4, 33.259619) (-28.361101, 7.4, 29.122868) (-15.980762, 4.8, 34.346159) (-11.040593, 4.8, 39.122868) (-17.037386, 7.4, 39.509619) (-24.20245, 4.8, 46.919873)
thicken "Thicken3" operation add thickness 0.05 both sides no extend neighbours yes toward (-0.8660254, 0, -0.5) faces at (6.108439, 4.8, 64.419873) (8.943376, 7.4, 54.509619) (6.279915, 7.4, 49.122868) (18.660254, 7.4, 54.346159) (22.76709, 7.4, 60.566243) (17.60363, 7.4, 59.509619) (10.438566, 7.4, 66.919873)
thicken "Thicken4" operation add thickness 0.05 both sides no extend neighbours yes toward (0, 0, 1) faces at (47.735027, 4.8, 42.5) (42.735027, 7.4, 47.5) (39.401694, 4.8, 50) (37.735027, 4.8, 36.666667) (41.06836, 4.8, 30) (42.735027, 7.4, 35) (52.735027, 4.8, 37.5)
thicken "Thicken5" operation add thickness 0.05 both sides no extend neighbours yes toward (0, 0, 1) faces at (52.735027, 7.4, 2.5) (42.735027, 7.4, 5) (39.401694, 4.8, 10) (37.735027, 4.8, -3.333333) (41.06836, 4.8, -10) (42.735027, 4.8, -5) (52.735027, 4.8, -2.5)
thicken "Thicken6" operation add thickness 0.05 both sides no extend neighbours yes toward (0, 0, 1) faces at (47.735027, 4.8, -37.5) (42.735027, 7.4, -35) (39.401694, 4.8, -30) (37.735027, 7.4, -43.333333) (41.06836, 4.8, -50) (42.735027, 7.4, -45) (52.735027, 4.8, -42.5)
body "Solid1"
